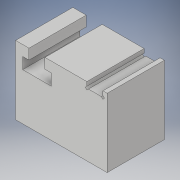
# Autodesk Inventor part: PiesaSuportCanale
Saved by Autodesk Inventor 2019 (Build 230136000, 136)
## iProperties
Created: 2020-03-10
Part Number: PiesaSuportCanale
Material: Generic
Document SubType Name: Modeling
Designer: Gabriel
Density: 1 g/cm^3
Appearance: Default
Author: Gabriel
Autodesk Inventor part; units mm, degrees
ref_plane "YZ Plane" through (0, 0, 0) normal (1, 0, 0) x (0, 1, 0)
ref_plane "XZ Plane" through (0, 0, 0) normal (0, 1, 0) x (-1, 0, 0)
ref_plane "XY Plane" through (0, 0, 0) normal (0, 0, 1) x (1, 0, 0)
sketch "Sketch1" plane through (0, 0, 0) normal (0, 0, 1) x (1, 0, 0)
  line L0 (-31.6809, 29.4017) -> (48.3191, 29.4017)
  line L1 (48.3191, 29.4017) -> (48.3191, -30.5983)
  line L2 (48.3191, -30.5983) -> (-31.6809, -30.5983)
  line L3 (-31.6809, -30.5983) -> (-31.6809, 29.4017)
  point P0 (0, 0)
  dimension "d0" = 80
  dimension "d1" = 60
  constraints: 8 end point, 2 parallel, 1 horizontal, 1 perpendicular
  measures "d0" distance of L0.start L0.end
  measures "d1" distance of L2.end L0.start
extrude "Extrusion1" add sketch "Sketch1" along normal blind 50
sketch "Sketch2" plane through (0, 0, 50) normal (0, 0, 1) x (1, 0, 0)
  line L0 (-19.9929, 29.4017) -> (-5.9929, 29.4017)
  line L1 (-5.9929, 29.4017) -> (-5.9929, 20.4017)
  line L2 (-5.9929, 20.4017) -> (-0.4929, 20.4017)
  line L3 (-0.4929, 20.4017) -> (-0.4929, 10.4017)
  line L4 (-0.4929, 10.4017) -> (-25.4929, 10.4017)
  line L5 (-25.4929, 10.4017) -> (-25.4929, 20.4017)
  line L6 (-25.4929, 20.4017) -> (-19.9929, 20.4017)
  line L7 (-19.9929, 20.4017) -> (-19.9929, 29.4017)
  line L8 (48.3191, 29.4017) -> (-31.6809, 29.4017) projected
  point P0 (0, 0)
  point P1 (-12.9929, 29.4017)
  dimension "d4" = 25
  dimension "d5" = 12.5
  dimension "d6" = 7
  dimension "d7" = 14
  dimension "d8" = 9
  dimension "d9" = 10
  constraints: 16 end point, 6 perpendicular, 3 point on line, 1 horizontal, 1 midpoint
  measures "d4" distance of L3.end L4.end
  measures "d5" distance from line of L5 point (-12.993, 29.402)
  measures "d6" distance from line of point (-12.993, 29.402) L7
  measures "d7" distance between parallel lines of L1 L7
  measures "d8" distance between parallel lines of L6 L0
  measures "d9" distance between parallel lines of L4 L6
extrude "Extrusion2" cut sketch "Sketch2" against normal blind 50
sketch "Sketch3" plane through (0, 0, 50) normal (0, 0, 1) x (1, 0, 0)
  line L0 (37.593, 29.4385) -> (44.593, 29.4385)
  line L1 (44.593, 29.4385) -> (44.593, 25.8997)
  line L2 (44.593, 25.8997) -> (46.0072, 24.4855)
  line L3 (46.0072, 24.4855) -> (44.593, 23.0713)
  line L4 (44.593, 23.0713) -> (43.2258, 24.4385)
  line L5 (43.2258, 24.4385) -> (37.593, 24.4385)
  line L6 (37.593, 29.4385) -> (37.593, 24.4385) construction
  line L7 (37.593, 29.4385) -> (30.593, 29.4385)
  line L8 (30.593, 29.4385) -> (30.593, 25.8997)
  line L9 (30.593, 25.8997) -> (29.1788, 24.4855)
  line L10 (29.1788, 24.4855) -> (30.593, 23.0713)
  line L11 (30.593, 23.0713) -> (31.9602, 24.4385)
  line L12 (31.9602, 24.4385) -> (37.593, 24.4385)
  point P0 (0, 0)
  point P1 (31.0916, 30.5867)
  dimension "d23" = 7
  dimension "d24" = 2
  dimension "d26" = 2
  dimension "d27" = 135
  dimension "d28" = 5
  constraints: 26 end point, 5 symmetric about line, 4 perpendicular, 1 coincident, 1 horizontal, 1 parallel
  measures "d23" distance of L0.end L0.start
  measures "d24" distance from line of L3 L1.end
  measures "d26" distance from line of L4 L2.end
  measures "d27" angle of L5 L4
  measures "d28" distance between parallel lines of L5 L0
extrude "Extrusion3" cut sketch "Sketch3" against normal blind 50
body "Solid1"
